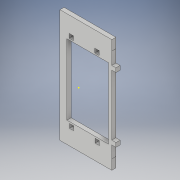
# Autodesk Inventor part: openslotforclamp
Saved by Autodesk Inventor 2019 (Build 230136000, 136)
## iProperties
Created: 2020-02-26
Part Number: openslotforclamp
Material: Generic
Document SubType Name: Modeling
Designer: Hp
Density: 1 g/cm^3
Appearance: Default
Author: Hp
Autodesk Inventor part; units mm, degrees
ref_plane "YZ Plane" through (0, 0, 0) normal (1, 0, 0) x (0, 1, 0)
ref_plane "XZ Plane" through (0, 0, 0) normal (0, 1, 0) x (-1, 0, 0)
ref_plane "XY Plane" through (0, 0, 0) normal (0, 0, 1) x (1, 0, 0)
sketch "Sketch1" plane through (0, 0, 0) normal (0, 0, 1) x (1, 0, 0)
  line L0 (-9.019, 23.22) -> (15.981, 23.22)
  line L1 (15.981, 23.22) -> (15.981, -21.78)
  line L2 (15.981, -21.78) -> (-9.019, -21.78)
  line L3 (-9.019, -21.78) -> (-9.019, 23.22)
  line L4 (-5.6447, 21.5683) -> (14.3553, 21.5683)
  line L5 (14.3553, 21.5683) -> (14.3553, -20.4317)
  line L6 (14.3553, -20.4317) -> (-5.6447, -20.4317)
  line L7 (-5.6447, -20.4317) -> (-5.6447, 21.5683)
  line L8 (17.9795, 15.2281) -> (17.9795, -13.9821)
  line L9 (17.9795, 15.2281) -> (15.9795, 15.2281)
  line L10 (15.9795, 15.2281) -> (15.9795, 17.2281)
  line L11 (15.9795, 17.2281) -> (17.9795, 17.2281)
  line L12 (17.9795, 17.2281) -> (17.9795, 15.2281)
  line L13 (17.9795, -13.9821) -> (15.9795, -13.9821)
  line L14 (15.9795, -13.9821) -> (15.9795, -15.9821)
  line L15 (15.9795, -15.9821) -> (17.9795, -15.9821)
  line L16 (17.9795, -15.9821) -> (17.9795, -13.9821)
  point P0 (0, 0)
  dimension "d0" = 25
  dimension "d2" = 20
  dimension "d4" = 29.2102
  dimension "d5" = 2
  dimension "d6" = 2
  dimension "d7" = 2
  dimension "d8" = 2
  constraints: 34 end point, 8 parallel, 4 horizontal, 4 perpendicular, 1 vertical
  measures "d0" distance of L1.end L2.end
  measures "d2" distance of L5.end L6.end
  measures "d4" distance of L8.start L8.end
  measures "d5" distance of L10.end L11.end
  measures "d6" distance of L9.end L10.end
  measures "d7" distance of L15.end L14.end
  measures "d8" distance of L14.end L13.end
extrude "Extrusion1" add sketch "Sketch1" along normal blind 2 contours L0 L1 L2 L3 | L11 L12 L9 L1 | L1 L13 L16 L15
sketch "Sketch2" plane through (0, 0, 2) normal (0, 0, 1) x (1, 0, 0)
  line L0 (-9.019, 23.22) -> (-9.019, -21.78) projected
  line L1 (-9.019, -21.78) -> (15.9746, -21.78)
  line L2 (15.9746, -21.78) -> (15.9746, -26.578)
  line L3 (15.9746, -26.578) -> (-9.019, -26.578)
  line L4 (-9.019, -26.578) -> (-9.019, -21.78)
  line L5 (-9.019, 23.22) -> (15.981, 23.22) projected
  line L6 (-9.019, 23.22) -> (15.9746, 23.22)
  line L7 (15.9746, 23.22) -> (15.9746, 27.9895)
  line L8 (15.9746, 27.9895) -> (-9.019, 27.9895)
  line L9 (-9.019, 27.9895) -> (-9.019, 23.22)
  point P0 (0, 0)
  constraints: 16 end point, 4 parallel, 2 horizontal, 2 perpendicular, 1 point on line
extrude "Extrusion2" add sketch "Sketch2" against normal blind 2
sketch "Sketch3" plane through (0, 0, 2) normal (0, 0, 1) x (1, 0, 0)
  line L0 (-5.6447, -20.4317) -> (14.3553, -20.4317) projected
  line L1 (14.3553, -20.4317) -> (14.3553, 21.5683) projected
  line L2 (-5.6447, -20.4317) -> (14.3553, -20.4317)
  line L3 (14.3553, -20.4317) -> (14.3553, -15.4317)
  line L4 (14.3553, -15.4317) -> (-5.6447, -15.4317)
  line L5 (-5.6447, -15.4317) -> (-5.6447, -20.4317)
  line L6 (-5.6447, 21.5683) -> (-5.6447, -20.4317) projected
  line L7 (-5.6447, 21.5683) -> (14.3553, 21.5683)
  line L8 (14.3553, 21.5683) -> (14.3553, 16.5683)
  line L9 (14.3553, 16.5683) -> (-5.6447, 16.5683)
  line L10 (-5.6447, 16.5683) -> (-5.6447, 21.5683)
  point P0 (0, 0)
  dimension "d13" = 5
  dimension "d14" = 5
  constraints: 16 end point, 4 parallel, 2 horizontal, 2 perpendicular, 2 point on line
  measures "d13" distance of L3.end L2.end
  measures "d14" distance of L7.end L8.end
extrude "Extrusion3" add sketch "Sketch3" against normal blind 2 contours L5 L4 L1 L0 | L6 L7 L1 L9
sketch "Sketch4" plane through (0, 0, 2) normal (0, 0, 1) x (1, 0, 0)
  point P0 (0, 0)
sketch "Sketch5" plane through (0, 0, 2) normal (0, 0, 1) x (1, 0, 0)
  line L0 (-5.6447, -15.4317) -> (14.3572, -15.4317)
  line L1 (14.3572, -15.4317) -> (14.3572, -16.4317)
  line L2 (14.3572, -16.4317) -> (-5.6447, -16.4317)
  line L3 (-5.6447, -16.4317) -> (-5.6447, -15.4317)
  line L4 (-5.6447, -15.4317) -> (-5.6447, 16.5683) projected
  line L5 (-5.6447, 16.5683) -> (14.3572, 16.5683)
  line L6 (14.3572, 16.5683) -> (14.3572, 17.5683)
  line L7 (14.3572, 17.5683) -> (-5.6447, 17.5683)
  line L8 (-5.6447, 17.5683) -> (-5.6447, 16.5683)
  point P0 (0, 0)
  dimension "d17" = 1
  dimension "d18" = 1
  constraints: 16 end point, 4 parallel, 2 horizontal, 2 perpendicular, 1 point on line
  measures "d17" distance of L0.end L1.end
  measures "d18" distance of L6.end L5.end
extrude "Extrusion4" cut sketch "Sketch5" against normal blind 2
sketch "Sketch6" plane through (0, 0, 2) normal (0, 0, 1) x (1, 0, 0)
  point P0 (0, 0)
sketch "Sketch7" plane through (0, 0, 2) normal (0, 0, 1) x (1, 0, 0)
  line L0 (-4.5311, 20.3235) -> (-2.5311, 20.3235)
  line L1 (-2.5311, 20.3235) -> (-2.5311, 18.3235)
  line L2 (-2.5311, 18.3235) -> (-4.5311, 18.3235)
  line L3 (-4.5311, 18.3235) -> (-4.5311, 20.3235)
  line L4 (-2.5311, 19.3235) -> (7.8219, 19.3235)
  line L5 (7.8219, 20.3235) -> (9.8242, 20.3235)
  line L6 (9.8242, 20.3235) -> (9.8242, 18.3235)
  line L7 (9.8242, 18.3235) -> (7.8219, 18.3235)
  line L8 (7.8219, 18.3235) -> (7.8219, 20.3235)
  point P0 (0, 0)
  dimension "d21" = 2
  dimension "d22" = 2
  dimension "d23" = 10.353
  constraints: 18 end point, 4 parallel, 3 horizontal, 2 perpendicular, 1 midpoint
  measures "d21" distance of L1.end L2.end
  measures "d22" distance of L0.end L1.end
  measures "d23" distance of L4.start L4.end
extrude "Extrusion5" cut sketch "Sketch7" against normal blind 10
sketch "Sketch8" plane through (0, 0, 2) normal (0, 0, 1) x (1, 0, 0)
  line L0 (14.3572, -16.4317) -> (-5.6447, -16.4317) projected
  line L1 (-4.3843, -16.4317) -> (-4.3843, -17.2017)
  line L2 (-4.3843, -17.2017) -> (-2.3843, -17.2017)
  line L3 (-2.3843, -17.2017) -> (-2.3843, -19.2017)
  line L4 (-2.3843, -19.2017) -> (-4.3843, -19.2017)
  line L5 (-4.3843, -19.2017) -> (-4.3843, -17.2017)
  line L6 (-2.3843, -18.2017) -> (7.9687, -18.2017)
  line L7 (7.9687, -17.2017) -> (9.9687, -17.2017)
  line L8 (9.9687, -17.2017) -> (9.9687, -19.2017)
  line L9 (9.9687, -19.2017) -> (7.9687, -19.2017)
  line L10 (7.9687, -19.2017) -> (7.9687, -17.2017)
  point P0 (0, 0)
  dimension "d26" = 0.77
  dimension "d27" = 2
  dimension "d28" = 2
  dimension "d29" = 10.353
  dimension "d30" = 2
  constraints: 20 end point, 4 parallel, 3 horizontal, 3 perpendicular, 1 midpoint, 1 point on line
  measures "d26" distance of L1.start L1.end
  measures "d27" distance of L3.end L4.end
  measures "d28" distance of L2.end L3.end
  measures "d29" distance of L6.start L6.end
  measures "d30" distance of L8.end L9.end
extrude "Extrusion6" cut sketch "Sketch8" against normal blind 10
sketch "Sketch9" plane through (0, 0, 2) normal (0, 0, 1) x (1, 0, 0)
  point P0 (0, 0)
body "Solid1"
